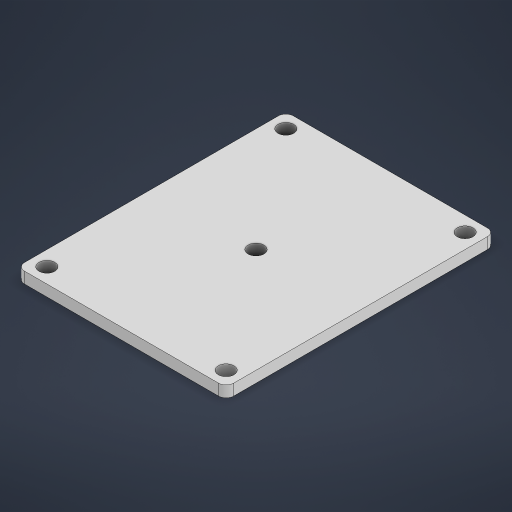
# Autodesk Inventor part: StageConnectionPlate
Saved by Autodesk Inventor 2024 (Build 280153000, 153)
## iProperties
Created: 2024-02-27
Part Number: StageConnectionPlate
Material: Generic
Document SubType Name: Modeling
Designer: avsar
Density: 1 g/cm^3
Appearance: Default
Author: avsar
Autodesk Inventor part; units mm, degrees
ref_plane "YZ Plane" through (0, 0, 0) normal (1, 0, 0) x (0, 1, 0)
ref_plane "XZ Plane" through (0, 0, 0) normal (0, 1, 0) x (-1, 0, 0)
ref_plane "XY Plane" through (0, 0, 0) normal (0, 0, 1) x (1, 0, 0)
sketch "Sketch1" plane through (0, 0, 0) normal (0, 1, 0) x (-1, 0, 0)
  line L0 (24, 32) -> (-24, 32) construction
  line L1 (-24, 32) -> (-24, -32) construction
  line L2 (-24, -32) -> (24, -32) construction
  line L3 (24, -32) -> (24, 32) construction
  line L4 (24, 32) -> (-24, -32) construction
  line L5 (-24, 32) -> (24, -32) construction
  line L6 (26, 36) -> (-26, 36)
  line L7 (-28, 34) -> (-28, -34)
  line L8 (-26, -36) -> (26, -36)
  line L9 (28, -34) -> (28, 34)
  arc A0 (26, -36) -> (28, -34) centre (26, -34) ccw
  arc A1 (28, 34) -> (26, 36) centre (26, 34) ccw
  arc A2 (-26, 36) -> (-28, 34) centre (-26, 34) ccw
  arc A3 (-28, -34) -> (-26, -36) centre (-26, -34) ccw
  circle A4 centre (24, -32) radius 2.1
  circle A5 centre (-24, -32) radius 2.1
  circle A6 centre (-24, 32) radius 2.1
  circle A7 centre (24, 32) radius 2.1
  circle A8 centre (0, 0) radius 2.1
  dimension "d0" = 48
  dimension "d1" = 64
  dimension "d2" = 4
  dimension "d3" = 2
  dimension "d4" = 4.2
  dimension "d5" = 4.2
  dimension "d6" = 4.2
  dimension "d7" = 4.2
  dimension "d8" = 4.2
  constraints: 20 end point, 9 centre point, 8 point on circle, 8 tangent, 5 coincident, 4 parallel, 3 equal radius, 2 midpoint, 2 perpendicular, 1 horizontal, 3 other
  measures "d0" distance of L2.end L1.end
  measures "d1" distance of L1.end L0.end
  measures "d2" distance between parallel lines of L3 L9
  measures "d3" radius of A0
  measures "d4" diameter of A4
  measures "d5" diameter of A5
  measures "d6" diameter of A6
  measures "d7" diameter of A7
  measures "d8" diameter of A8
extrude "Extrusion1" add sketch "Sketch1" along normal blind 3
body "Solid1"
